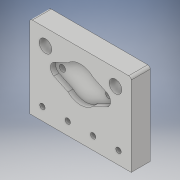
# Autodesk Inventor part: End_atrail
Saved by Autodesk Inventor 2019 (Build 230136000, 136)
## iProperties
Created: 2021-06-20
Part Number: End_atrail
Material: Generic
Document SubType Name: Modeling
Designer: 91742
Density: 1 g/cm^3
Appearance: Default
Author: 91742
Autodesk Inventor part; units mm, degrees
ref_plane "YZ Plane" through (0, 0, 0) normal (1, 0, 0) x (0, 1, 0)
ref_plane "XZ Plane" through (0, 0, 0) normal (0, 1, 0) x (-1, 0, 0)
ref_plane "XY Plane" through (0, 0, 0) normal (0, 0, 1) x (1, 0, 0)
sketch "Sketch1" plane through (0, 0, 0) normal (0, 0, 1) x (1, 0, 0)
  line L0 (38, 55) -> (0, 55)
  line L1 (-38, 55) -> (0, 55)
  arc A0 (-38, 55) -> (-40, 53) centre (-38, 53) ccw
  arc A1 (40, 53) -> (38, 55) centre (38, 53) ccw
  circle A2 centre (27.6, 42.5) radius 5
  circle A3 centre (-27.6, 42.5) radius 5
  line L2 (-40, 2) -> (-40, 2)
  line L3 (40, 2) -> (40, 2)
  line L4 (-40, 53) -> (-40, 0)
  line L5 (40, 0) -> (40, 53)
  line L6 (-40, 0) -> (-40, -10)
  line L7 (-40, -10) -> (40, -10)
  line L8 (40, -10) -> (40, 0)
  circle A4 centre (30, 0) radius 2.1
  circle A5 centre (-30, 0) radius 2.1
  circle A6 centre (-10, 0) radius 2.1
  circle A7 centre (10, 0) radius 2.1
  point P0 (0, 0)
  point P1 (40, 55)
  dimension "d0" = 2
  dimension "d2" = 10
  dimension "d3" = 10
  dimension "d4" = 4.2
  dimension "d5" = 4.2
  dimension "d6" = 4.2
  dimension "d7" = 4.2
  dimension "d8" = 52.5
  constraints: 18 end point, 8 centre point, 5 vertical, 4 point on circle, 2 horizontal, 2 point on line, 2 tangent, 1 equal radius, 1 perpendicular
  measures "d0" radius of A0
  measures "d2" diameter of A2
  measures "d3" distance of L4.end L7.start
  measures "d4" diameter of A4
  measures "d5" diameter of A5
  measures "d6" diameter of A6
  measures "d7" diameter of A7
  measures "d8" distance from line of L7 A3.centre
extrude "Extrusion1" add sketch "Sketch1" along normal blind 15
sketch "Sketch6" plane through (0, 0, 15) normal (0, 0, 1) x (1, 0, 0)
  circle A0 centre (-18.25, 30) radius 2.5
  circle A1 centre (0, 30) radius 13.5
  line L0 (-18.25, 30) -> (-12.75, 30) construction
  line L1 (-18.25, 30) -> (-12.75, 30) construction
  arc A2 (-21, 34.7631) -> (-21, 25.2369) centre (-18.25, 30) ccw
  line L2 (-21, 34.7631) -> (-1.6262, 34.7631) construction
  line L3 (-21, 25.2369) -> (-9.8237, 20.0252)
  line L4 (-21, 25.2369) -> (-7.9961, 25.2369) construction
  line L5 (-21, 34.7631) -> (-9.8237, 39.9748)
  circle A3 centre (18.25, 30) radius 2.5
  line L6 (18.25, 30) -> (12.75, 30) construction
  line L7 (18.25, 30) -> (12.75, 30) construction
  arc A4 (21, 25.2369) -> (21, 34.7631) centre (18.25, 30) ccw
  line L8 (21, 25.2369) -> (9.8237, 20.0252)
  line L9 (21, 25.2369) -> (7.9961, 25.2369) construction
  line L10 (21, 34.7631) -> (9.8237, 39.9748)
  line L11 (21, 34.7631) -> (1.6262, 34.7631) construction
  arc A5 (-9.8237, 20.0252) -> (9.8237, 20.0252) centre (0, 30) ccw
  arc A6 (9.8237, 39.9748) -> (-9.8237, 39.9748) centre (0, 30) ccw
  point P0 (0, 0)
  dimension "d39" = 5
  dimension "d40" = 27
  dimension "d41" = 25
  constraints: 24 end point, 8 point on circle, 7 centre point, 5 coincident, 4 horizontal
  measures "d39" diameter of A0
  measures "d40" diameter of A1
  measures "d41" angle of L3 L4
extrude "Extrusion5" cut sketch "Sketch6" against normal blind 4
sketch "Sketch7" plane through (0, 30, 15) normal (0, 0, 1) x (1, 0, 0)
  circle A0 centre (0, 0) radius 13.5
  point P0 (0, -30)
  dimension "d44" = 27
  constraints: 1 centre point
  measures "d44" diameter of A0
extrude "Extrusion6" cut sketch "Sketch7" against normal blind 4
sketch "Sketch8" plane through (-18.25, 30, 15) normal (0, 0, 1) x (1, 0, 0)
  circle A0 centre (0, 0) radius 2.5
  point P0 (18.25, -30)
  dimension "d47" = 5
  constraints: 1 centre point
  measures "d47" diameter of A0
extrude "Extrusion7" cut sketch "Sketch8" against normal blind 20
sketch "Sketch9" plane through (18.25, 30, 15) normal (0, 0, 1) x (1, 0, 0)
  circle A0 centre (0, 0) radius 2.5
  point P0 (-18.25, -30)
  dimension "d50" = 5
  constraints: 1 centre point
  measures "d50" diameter of A0
extrude "Extrusion8" cut sketch "Sketch9" against normal blind 20
body "Solid1"
